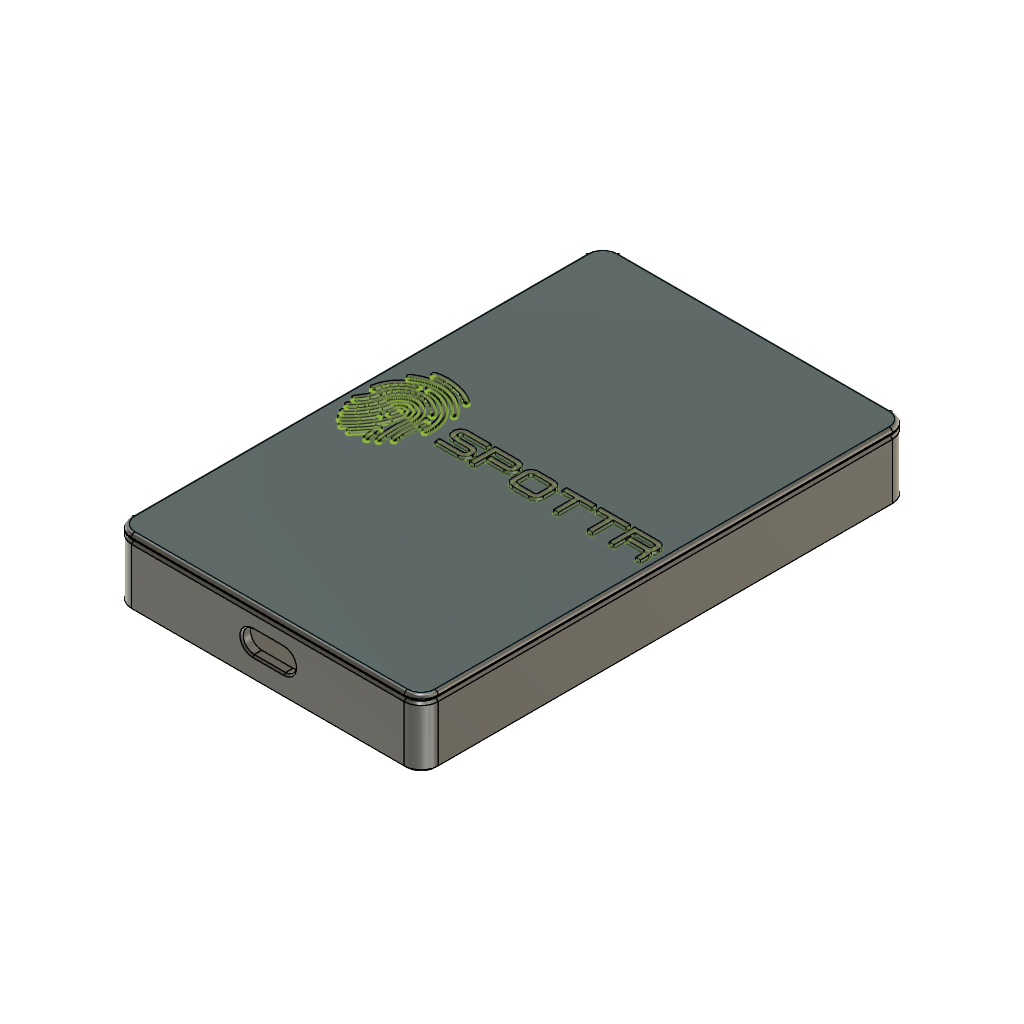
Spottr (Autodesk Fusion 360 archive; units mm, degrees)
design "CASE_BODY"
Autodesk Fusion 360 part; units mm, degrees
note: some values were not read from the file. Set by a fixed rule: which sketch regions a step uses.
(part 1 of 5)
sketch "CARD_SKETCH" plane through (0, 0, 0) normal (0, 0, 1) x (1, 0, 0)
  line L0 (0, 0) -> (54, 0)
  line L1 (54, 0) -> (54, 86)
  line L2 (54, 86) -> (0, 86)
  line L3 (0, 86) -> (0, 0)
  dimension "d3" = 54
  dimension "d4" = 86
  constraint horizontal L0
  constraint vertical L1
  constraint horizontal L2
  constraint vertical L3
  constraint coincident L0.start L3.end
  measures "d3" distance of L0.start L0.end
  measures "d4" distance of L0.start L2.end
extrude "Extrude1" add sketch "CARD_SKETCH" along normal blind 11.9 contours L0 L1 L2 L3 picked at (18, 28.666667) makes body 1
fillet "Fillet1" radius 3 4 edges at (54, 0, 5.95) (0, 0, 5.95) (54, 86, 5.95) (0, 86, 5.95) on bodies 1
ref_plane "WorkPlane1" through (27, 43, 10.7) normal (0, 0, -1) x (-1, 0, 0)
split "Split1" by plane through (27, 43, 10.7) normal (0, 0, -1) bodies 1 makes body 2 at (18, 56.333333, 0)
sketch "CARD_HOLLOW_SKETCH" plane through (0, 0, 10.7) normal (0, 0, 1) x (-1, 0, 0)
  arc A0 (0, -3) -> (-3, 0) centre (-3, -3) ccw
  line L0 (-3, 0) -> (-51, 0)
  arc A1 (-51, 0) -> (-54, -3) centre (-51, -3) ccw
  line L1 (-54, -3) -> (-54, -83)
  arc A2 (-54, -83) -> (-51, -86) centre (-51, -83) ccw
  line L2 (-51, -86) -> (-3, -86)
  arc A3 (-3, -86) -> (0, -83) centre (-3, -83) ccw
  line L3 (0, -83) -> (0, -3)
  line L4 (-54, -83) -> (-54, -3)
  arc A4 (-54, -83) -> (-51, -86) centre (-51, -83) ccw
  line L5 (-3, -86) -> (-51, -86)
  arc A5 (-3, -86) -> (0, -83) centre (-3, -83) ccw
  line L6 (0, -3) -> (0, -83)
  arc A6 (-51, 0) -> (-54, -3) centre (-51, -3) ccw
  line L7 (-51, 0) -> (-3, 0)
  arc A7 (0, -3) -> (-3, 0) centre (-3, -3) ccw
  line L8 (-51, -84.4) -> (-3, -84.4)
  arc A8 (-3, -84.4) -> (-1.6, -83) centre (-3, -83) ccw
  line L9 (-1.6, -83) -> (-1.6, -3)
  arc A9 (-1.6, -3) -> (-3, -1.6) centre (-3, -3) ccw
  line L10 (-3, -1.6) -> (-51, -1.6)
  arc A10 (-51, -1.6) -> (-52.4, -3) centre (-51, -3) ccw
  line L11 (-52.4, -3) -> (-52.4, -83)
  arc A11 (-52.4, -83) -> (-51, -84.4) centre (-51, -83) ccw
extrude "Extrude2" cut sketch "CARD_HOLLOW_SKETCH" against normal blind 9.5 contours L8 A8 L9 A9 L10 A10 L11 A11 picked at (-35.466667, -29.666667) bodies 2
sketch "LID_PLUG_SKETCH" plane through (0, 0, 10.7) normal (0, 0, -1) x (1, 0, 0)
  arc A0 (3, 0) -> (0, -3) centre (3, -3) ccw
  line L0 (0, -3) -> (0, -83)
  arc A1 (0, -83) -> (3, -86) centre (3, -83) ccw
  line L1 (3, -86) -> (51, -86)
  arc A2 (51, -86) -> (54, -83) centre (51, -83) ccw
  line L2 (54, -83) -> (54, -3)
  arc A3 (54, -3) -> (51, 0) centre (51, -3) ccw
  line L3 (51, 0) -> (3, 0)
  line L4 (3, -84.2) -> (51, -84.2)
  arc A4 (51, -84.2) -> (52.2, -83) centre (51, -83) ccw
  line L5 (52.2, -83) -> (52.2, -3)
  arc A5 (52.2, -3) -> (51, -1.8) centre (51, -3) ccw
  line L6 (51, -1.8) -> (3, -1.8)
  arc A6 (3, -1.8) -> (1.8, -3) centre (3, -3) ccw
  line L7 (1.8, -3) -> (1.8, -83)
  arc A7 (1.8, -83) -> (3, -84.2) centre (3, -83) ccw
  line L8 (51.4, -83) -> (51.4, -3)
  arc A8 (51.4, -3) -> (51, -2.6) centre (51, -3) ccw
  line L9 (51, -2.6) -> (3, -2.6)
  arc A9 (3, -2.6) -> (2.6, -3) centre (3, -3) ccw
  line L10 (2.6, -3) -> (2.6, -83)
  arc A10 (2.6, -83) -> (3, -83.4) centre (3, -83) ccw
  line L11 (3, -83.4) -> (51, -83.4)
  arc A11 (51, -83.4) -> (51.4, -83) centre (51, -83) ccw
extrude "Extrude3" add sketch "LID_PLUG_SKETCH" along normal blind 1 contours L4 A4 L5 A5 L6 A6 L7 A7 picked at (51.933333, -56.333333) bodies 1
ref_plane "WorkPlane3" through (27, 43, 5.35) normal (0, 1, 0) x (-1, 0, 0)
chamfer "Chamfer1" distance 0.5 angle 45 1 faces at (18, 56.333333, 0) tangent chain off on bodies 2
chamfer "Chamfer3" distance 0.4 angle 45 8 edges at (0, 43, 10.7) (0.87868, 85.12132, 10.7) (27, 86, 10.7) (53.12132, 85.12132, 10.7) (54, 43, 10.7) (53.12132, 0.87868, 10.7) (27, 0, 10.7) (0.87868, 0.87868, 10.7) tangent chain off on bodies 2
fillet "Fillet2" radius 0.6 1 faces at (18, 56.333333, 11.9) on bodies 1
chamfer "Chamfer4" distance 0.4 angle 45 8 edges at (0, 43, 10.7) (0.87868, 85.12132, 10.7) (27, 86, 10.7) (53.12132, 85.12132, 10.7) (54, 43, 10.7) (53.12132, 0.87868, 10.7) (27, 0, 10.7) (0.87868, 0.87868, 10.7) tangent chain off on bodies 1
sketch "LID_LOGO_SPOTTR_SKETCH" plane through (0, 0, 11.9) normal (0, 0, 1) x (-1, 0, 0)
  arc A0 (-3, -85.4) -> (-0.6, -83) centre (-3, -83) ccw
  line L0 (-0.6, -83) -> (-0.6, -3)
  arc A1 (-0.6, -3) -> (-3, -0.6) centre (-3, -3) ccw
  line L1 (-3, -0.6) -> (-51, -0.6)
  arc A2 (-51, -0.6) -> (-53.4, -3) centre (-51, -3) ccw
  line L2 (-53.4, -3) -> (-53.4, -83)
  arc A3 (-53.4, -83) -> (-51, -85.4) centre (-51, -83) ccw
  line L3 (-51, -85.4) -> (-3, -85.4)
  spline S0 degree 3 poles (-5.943652, -50.073493) (-6.506523, -50.208843) (-7.077484, -50.282586) (-7.656535, -50.294098) knots 0 0 0 0 1 1 1 1
  spline S1 degree 3 poles (-7.656535, -50.294098) (-8.235274, -50.305922) (-8.808724, -50.255515) (-9.376574, -50.142879) knots 0 0 0 0 1 1 1 1
  spline S2 degree 3 poles (-9.376574, -50.142879) (-9.948468, -50.05109) (-10.504182, -49.89956) (-11.043407, -49.688288) knots 0 0 0 0 1 1 1 1
  spline S3 degree 3 poles (-11.043407, -49.688288) (-11.58294, -49.476706) (-12.093539, -49.210362) (-12.575511, -48.888943) knots 0 0 0 0 1 1 1 1
  spline S4 degree 3 poles (-12.575511, -48.888943) (-12.594491, -48.875253) (-12.614716, -48.86374) (-12.635874, -48.854095) knots 0 0 0 0 1 1 1 1
  spline S5 degree 3 poles (-12.635874, -48.854095) (-12.657343, -48.844138) (-12.679435, -48.83667) (-12.702149, -48.831381) knots 0 0 0 0 1 1 1 1
  spline S6 degree 3 poles (-12.702149, -48.831381) (-12.724863, -48.826091) (-12.748199, -48.823291) (-12.771536, -48.822668) knots 0 0 0 0 1 1 1 1
  spline S7 degree 3 poles (-12.771536, -48.822668) (-12.794872, -48.821737) (-12.818208, -48.823599) (-12.841233, -48.827647) knots 0 0 0 0 1 1 1 1
  spline S8 degree 3 poles (-12.841233, -48.827647) (-12.864258, -48.831383) (-12.886661, -48.837604) (-12.908753, -48.846316) knots 0 0 0 0 1 1 1 1
  spline S9 degree 3 poles (-12.908753, -48.846316) (-12.930533, -48.854717) (-12.951069, -48.865296) (-12.970983, -48.877742) knots 0 0 0 0 1 1 1 1
  spline S10 degree 3 poles (-12.970983, -48.877742) (-12.990585, -48.890499) (-13.008943, -48.905123) (-13.025745, -48.921303) knots 0 0 0 0 1 1 1 1
  spline S11 degree 3 poles (-13.025745, -48.921303) (-13.042547, -48.937483) (-13.057794, -48.955218) (-13.070862, -48.974821) knots 0 0 0 0 1 1 1 1
  spline S12 degree 3 poles (-13.070862, -48.974821) (-13.084242, -48.994112) (-13.095443, -49.014337) (-13.104778, -49.035806) knots 0 0 0 0 1 1 1 1
  spline S13 degree 3 poles (-13.104778, -49.035806) (-13.114112, -49.057587) (-13.120957, -49.079679) (-13.125625, -49.102704) knots 0 0 0 0 1 1 1 1
  spline S14 degree 3 poles (-13.125625, -49.102704) (-13.130603, -49.125729) (-13.133089, -49.148754) (-13.133089, -49.172401) knots 0 0 0 0 1 1 1 1
  spline S15 degree 3 poles (-13.133089, -49.172401) (-13.133407, -49.195738) (-13.131224, -49.219074) (-13.126557, -49.242099) knots 0 0 0 0 1 1 1 1
  spline S16 degree 3 poles (-13.126557, -49.242099) (-13.1222, -49.265124) (-13.115355, -49.287216) (-13.106643, -49.308996) knots 0 0 0 0 1 1 1 1
  spline S17 degree 3 poles (-13.106643, -49.308996) (-13.09762, -49.330777) (-13.086418, -49.351313) (-13.073661, -49.370604) knots 0 0 0 0 1 1 1 1
  spline S18 degree 3 poles (-13.073661, -49.370604) (-13.060593, -49.390207) (-13.045658, -49.408253) (-13.028856, -49.424744) knots 0 0 0 0 1 1 1 1
  spline S19 degree 3 poles (-13.028856, -49.424744) (-13.012365, -49.441235) (-12.994318, -49.455859) (-12.974716, -49.468616) knots 0 0 0 0 1 1 1 1
  spline S20 degree 3 poles (-12.974716, -49.468616) (-12.451361, -49.81866) (-11.896891, -50.108964) (-11.310995, -50.339526) knots 0 0 0 0 1 1 1 1
  spline S21 degree 3 poles (-11.310995, -50.339526) (-10.725099, -50.570088) (-10.121779, -50.73562) (-9.500411, -50.836122) knots 0 0 0 0 1 1 1 1
  spline S22 degree 3 poles (-9.500411, -50.836122) (-8.882467, -50.957471) (-8.258611, -51.011611) (-7.629154, -50.997609) knots 0 0 0 0 1 1 1 1
  spline S23 degree 3 poles (-7.629154, -50.997609) (-6.999386, -50.983918) (-6.378641, -50.902708) (-5.766608, -50.754289) knots 0 0 0 0 1 1 1 1
  spline S24 degree 3 poles (-5.766608, -50.754289) (-5.743583, -50.749) (-5.721492, -50.741532) (-5.700022, -50.731887) knots 0 0 0 0 1 1 1 1
  spline S25 degree 3 poles (-5.700022, -50.731887) (-5.678864, -50.722241) (-5.658639, -50.710417) (-5.639348, -50.696415) knots 0 0 0 0 1 1 1 1
  spline S26 degree 3 poles (-5.639348, -50.696415) (-5.620368, -50.682725) (-5.602944, -50.667167) (-5.587075, -50.650054) knots 0 0 0 0 1 1 1 1
  spline S27 degree 3 poles (-5.587075, -50.650054) (-5.570894, -50.63263) (-5.556893, -50.613961) (-5.544758, -50.593736) knots 0 0 0 0 1 1 1 1
  spline S28 degree 3 poles (-5.544758, -50.593736) (-5.532623, -50.573511) (-5.522666, -50.552353) (-5.514577, -50.530261) knots 0 0 0 0 1 1 1 1
  spline S29 degree 3 poles (-5.514577, -50.530261) (-5.506487, -50.508169) (-5.500887, -50.485456) (-5.497464, -50.462119) knots 0 0 0 0 1 1 1 1
  spline S30 degree 3 poles (-5.497464, -50.462119) (-5.494038, -50.438783) (-5.493106, -50.415447) (-5.494349, -50.39211) knots 0 0 0 0 1 1 1 1
  spline S31 degree 3 poles (-5.494349, -50.39211) (-5.495592, -50.368463) (-5.499327, -50.345438) (-5.505239, -50.322724) knots 0 0 0 0 1 1 1 1
  spline S32 degree 3 poles (-5.505239, -50.322724) (-5.51115, -50.299699) (-5.519241, -50.277918) (-5.529509, -50.25676) knots 0 0 0 0 1 1 1 1
  spline S33 degree 3 poles (-5.529509, -50.25676) (-5.539777, -50.235602) (-5.552223, -50.215688) (-5.566536, -50.197019) knots 0 0 0 0 1 1 1 1
  spline S34 degree 3 poles (-5.566536, -50.197019) (-5.580849, -50.17835) (-5.596717, -50.161237) (-5.614454, -50.145991) knots 0 0 0 0 1 1 1 1
  spline S35 degree 3 poles (-5.614454, -50.145991) (-5.632189, -50.130433) (-5.651169, -50.116742) (-5.671705, -50.10523) knots 0 0 0 0 1 1 1 1
  spline S36 degree 3 poles (-5.671705, -50.10523) (-5.692241, -50.093717) (-5.713711, -50.084072) (-5.735802, -50.076915) knots 0 0 0 0 1 1 1 1
  spline S37 degree 3 poles (-5.735802, -50.076915) (-5.758204, -50.069452) (-5.78123, -50.064469) (-5.804566, -50.061669) knots 0 0 0 0 1 1 1 1
  spline S38 degree 3 poles (-5.804566, -50.061669) (-5.827902, -50.059184) (-5.851238, -50.058555) (-5.874575, -50.060738) knots 0 0 0 0 1 1 1 1
  spline S39 degree 3 poles (-5.874575, -50.060738) (-5.897911, -50.062602) (-5.920936, -50.066958) (-5.943652, -50.073493) knots 0 0 0 0 1 1 1 1
  spline S40 degree 3 poles (-4.178186, -47.601092) (-4.26593, -47.6655) (-4.35523, -47.728042) (-4.446086, -47.788094) knots 0 0 0 0 1 1 1 1
  spline S41 degree 3 poles (-4.446086, -47.788094) (-4.536942, -47.848146) (-4.629354, -47.905708) (-4.723321, -47.961093) knots 0 0 0 0 1 1 1 1
  spline S42 degree 3 poles (-4.723321, -47.961093) (-4.816977, -48.016478) (-4.912189, -48.069685) (-5.008646, -48.120091) knots 0 0 0 0 1 1 1 1
  spline S43 degree 3 poles (-5.008646, -48.120091) (-5.105102, -48.170809) (-5.202804, -48.218726) (-5.30175, -48.264465) knots 0 0 0 0 1 1 1 1
  spline S44 degree 3 poles (-5.30175, -48.264465) (-5.400695, -48.309893) (-5.500574, -48.353143) (-5.601698, -48.393592) knots 0 0 0 0 1 1 1 1
  spline S45 degree 3 poles (-5.601698, -48.393592) (-5.702822, -48.434042) (-5.804879, -48.472002) (-5.90787, -48.507473) knots 0 0 0 0 1 1 1 1
  spline S46 degree 3 poles (-5.90787, -48.507473) (-6.010861, -48.542944) (-6.114785, -48.575615) (-6.219332, -48.605797) knots 0 0 0 0 1 1 1 1
  spline S47 degree 3 poles (-6.219332, -48.605797) (-6.323878, -48.635667) (-6.429358, -48.663048) (-6.53546, -48.68794) knots 0 0 0 0 1 1 1 1
  spline S48 degree 3 poles (-6.53546, -48.68794) (-6.641563, -48.712521) (-6.747976, -48.734613) (-6.855322, -48.753904) knots 0 0 0 0 1 1 1 1
  spline S49 degree 3 poles (-6.855322, -48.753904) (-6.962358, -48.773507) (-7.070016, -48.789998) (-7.177985, -48.803688) knots 0 0 0 0 1 1 1 1
  spline S50 degree 3 poles (-7.177985, -48.803688) (-7.285954, -48.81769) (-7.394235, -48.828891) (-7.502827, -48.837292) knots 0 0 0 0 1 1 1 1
  spline S51 degree 3 poles (-7.502827, -48.837292) (-7.611418, -48.845694) (-7.720009, -48.851294) (-7.828912, -48.854095) knots 0 0 0 0 1 1 1 1
  spline S52 degree 3 poles (-7.828912, -48.854095) (-7.937815, -48.856897) (-8.046406, -48.857209) (-8.155309, -48.854413) knots 0 0 0 0 1 1 1 1
  spline S53 degree 3 poles (-8.155309, -48.854413) (-8.264211, -48.851929) (-8.372803, -48.846323) (-8.481394, -48.838233) knots 0 0 0 0 1 1 1 1
  spline S54 degree 3 poles (-8.481394, -48.838233) (-8.589986, -48.830143) (-8.698266, -48.818942) (-8.806235, -48.805562) knots 0 0 0 0 1 1 1 1
  spline S55 degree 3 poles (-8.806235, -48.805562) (-8.914204, -48.791872) (-9.021862, -48.775381) (-9.129209, -48.75609) knots 0 0 0 0 1 1 1 1
  spline S56 degree 3 poles (-9.129209, -48.75609) (-9.236245, -48.737109) (-9.342969, -48.715329) (-9.449072, -48.690748) knots 0 0 0 0 1 1 1 1
  spline S57 degree 3 poles (-9.449072, -48.690748) (-9.555174, -48.666167) (-9.660343, -48.639097) (-9.7652, -48.609227) knots 0 0 0 0 1 1 1 1
  spline S58 degree 3 poles (-9.7652, -48.609227) (-9.869747, -48.579356) (-9.973671, -48.546685) (-10.076662, -48.511525) knots 0 0 0 0 1 1 1 1
  spline S59 degree 3 poles (-10.076662, -48.511525) (-10.179652, -48.476365) (-10.28171, -48.438716) (-10.382834, -48.398267) knots 0 0 0 0 1 1 1 1
  spline S60 degree 3 poles (-10.382834, -48.398267) (-10.483957, -48.357817) (-10.584148, -48.31519) (-10.683094, -48.269762) knots 0 0 0 0 1 1 1 1
  spline S61 degree 3 poles (-10.683094, -48.269762) (-10.782039, -48.224334) (-10.879741, -48.176417) (-10.976197, -48.12601) knots 0 0 0 0 1 1 1 1
  spline S62 degree 3 poles (-10.976197, -48.12601) (-11.072965, -48.075604) (-11.167866, -48.022708) (-11.261833, -47.967635) knots 0 0 0 0 1 1 1 1
  spline S63 degree 3 poles (-11.261833, -47.967635) (-11.355801, -47.91225) (-11.448212, -47.854687) (-11.539068, -47.794946) knots 0 0 0 0 1 1 1 1
  spline S64 degree 3 poles (-11.539068, -47.794946) (-11.629924, -47.734894) (-11.719224, -47.672664) (-11.80728, -47.608256) knots 0 0 0 0 1 1 1 1
  spline S65 degree 3 poles (-11.80728, -47.608256) (-11.895024, -47.543848) (-11.980901, -47.477262) (-12.065534, -47.408498) knots 0 0 0 0 1 1 1 1
  spline S66 degree 3 poles (-12.065534, -47.408498) (-12.149856, -47.339733) (-12.232311, -47.268791) (-12.31321, -47.195671) knots 0 0 0 0 1 1 1 1
  spline S67 degree 3 poles (-12.31321, -47.195671) (-12.394109, -47.122862) (-12.473141, -47.047874) (-12.549995, -46.970709) knots 0 0 0 0 1 1 1 1
  spline S68 degree 3 poles (-12.549995, -46.970709) (-12.627161, -46.893855) (-12.702148, -46.814823) (-12.775268, -46.733924) knots 0 0 0 0 1 1 1 1
  spline S69 degree 3 poles (-12.775268, -46.733924) (-12.848077, -46.653336) (-12.91902, -46.57057) (-12.988095, -46.486248) knots 0 0 0 0 1 1 1 1
  spline S70 degree 3 poles (-12.988095, -46.486248) (-13.056859, -46.401615) (-13.123445, -46.315738) (-13.187853, -46.227682) knots 0 0 0 0 1 1 1 1
  spline S71 degree 3 poles (-13.187853, -46.227682) (-13.252573, -46.139938) (-13.314803, -46.050638) (-13.374544, -45.959782) knots 0 0 0 0 1 1 1 1
  spline S72 degree 3 poles (-13.374544, -45.959782) (-13.401614, -45.923066) (-13.434596, -45.893196) (-13.473489, -45.869548) knots 0 0 0 0 1 1 1 1
  spline S73 degree 3 poles (-13.473489, -45.869548) (-13.512072, -45.845901) (-13.553766, -45.830343) (-13.598572, -45.822876) knots 0 0 0 0 1 1 1 1
  spline S74 degree 3 poles (-13.598572, -45.822876) (-13.643377, -45.815413) (-13.687872, -45.816344) (-13.732366, -45.826301) knots 0 0 0 0 1 1 1 1
  spline S75 degree 3 poles (-13.732366, -45.826301) (-13.77655, -45.835946) (-13.81731, -45.853682) (-13.85496, -45.879508) knots 0 0 0 0 1 1 1 1
  spline S76 degree 3 poles (-13.85496, -45.879508) (-13.892298, -45.905022) (-13.923724, -45.936759) (-13.948927, -45.97472) knots 0 0 0 0 1 1 1 1
  spline S77 degree 3 poles (-13.948927, -45.97472) (-13.97413, -46.012369) (-13.991244, -46.053441) (-14.000578, -46.097935) knots 0 0 0 0 1 1 1 1
  spline S78 degree 3 poles (-14.000578, -46.097935) (-14.009913, -46.14243) (-14.010535, -46.187235) (-14.002752, -46.23173) knots 0 0 0 0 1 1 1 1
  spline S79 degree 3 poles (-14.002752, -46.23173) (-13.994663, -46.276535) (-13.978794, -46.318229) (-13.954524, -46.356812) knots 0 0 0 0 1 1 1 1
  spline S80 degree 3 poles (-13.954524, -46.356812) (-13.888249, -46.457314) (-13.819174, -46.555948) (-13.747609, -46.653027) knots 0 0 0 0 1 1 1 1
  spline S81 degree 3 poles (-13.747609, -46.653027) (-13.676045, -46.750106) (-13.601991, -46.845318) (-13.525759, -46.938663) knots 0 0 0 0 1 1 1 1
  spline S82 degree 3 poles (-13.525759, -46.938663) (-13.449527, -47.032008) (-13.370806, -47.123175) (-13.289907, -47.212475) knots 0 0 0 0 1 1 1 1
  spline S83 degree 3 poles (-13.289907, -47.212475) (-13.209008, -47.302087) (-13.125931, -47.389209) (-13.040365, -47.474153) knots 0 0 0 0 1 1 1 1
  spline S84 degree 3 poles (-13.040365, -47.474153) (-12.955109, -47.559408) (-12.867676, -47.642174) (-12.778065, -47.723073) knots 0 0 0 0 1 1 1 1
  spline S85 degree 3 poles (-12.778065, -47.723073) (-12.688765, -47.803661) (-12.596975, -47.882071) (-12.50363, -47.957991) knots 0 0 0 0 1 1 1 1
  spline S86 degree 3 poles (-12.50363, -47.957991) (-12.409974, -48.034223) (-12.314762, -48.107655) (-12.217683, -48.178908) knots 0 0 0 0 1 1 1 1
  spline S87 degree 3 poles (-12.217683, -48.178908) (-12.120293, -48.250162) (-12.021347, -48.318926) (-11.920535, -48.385201) knots 0 0 0 0 1 1 1 1
  spline S88 degree 3 poles (-11.920535, -48.385201) (-11.820034, -48.451165) (-11.717665, -48.51495) (-11.613741, -48.575936) knots 0 0 0 0 1 1 1 1
  spline S89 degree 3 poles (-11.613741, -48.575936) (-11.509816, -48.636921) (-11.404648, -48.695418) (-11.297612, -48.750802) knots 0 0 0 0 1 1 1 1
  spline S90 degree 3 poles (-11.297612, -48.750802) (-11.190887, -48.806498) (-11.082607, -48.859705) (-10.973082, -48.9098) knots 0 0 0 0 1 1 1 1
  spline S91 degree 3 poles (-10.973082, -48.9098) (-10.863557, -48.959895) (-10.752788, -49.007501) (-10.640774, -49.051996) knots 0 0 0 0 1 1 1 1
  spline S92 degree 3 poles (-10.640774, -49.051996) (-10.529071, -49.09649) (-10.415812, -49.138185) (-10.301931, -49.177078) knots 0 0 0 0 1 1 1 1
  spline S93 degree 3 poles (-10.301931, -49.177078) (-10.187739, -49.215972) (-10.072924, -49.252066) (-9.957176, -49.285047) knots 0 0 0 0 1 1 1 1
  spline S94 degree 3 poles (-9.957176, -49.285047) (-9.841117, -49.318029) (-9.724747, -49.348211) (-9.607132, -49.375281) knots 0 0 0 0 1 1 1 1
  spline S95 degree 3 poles (-9.607132, -49.375281) (-9.489829, -49.402351) (-9.371903, -49.426621) (-9.253354, -49.447779) knots 0 0 0 0 1 1 1 1
  spline S96 degree 3 poles (-9.253354, -49.447779) (-9.134495, -49.468937) (-9.015636, -49.486984) (-8.896154, -49.50223) knots 0 0 0 0 1 1 1 1
  spline S97 degree 3 poles (-8.896154, -49.50223) (-8.776672, -49.517477) (-8.656568, -49.529612) (-8.536464, -49.538635) knots 0 0 0 0 1 1 1 1
  spline S98 degree 3 poles (-8.536464, -49.538635) (-8.41636, -49.547658) (-8.296256, -49.55357) (-8.17553, -49.556682) knots 0 0 0 0 1 1 1 1
  spline S99 degree 3 poles (-8.17553, -49.556682) (-8.055115, -49.559484) (-7.9347, -49.559484) (-7.814284, -49.556363) knots 0 0 0 0 1 1 1 1
  spline S100 degree 3 poles (-7.814284, -49.556363) (-7.693869, -49.553249) (-7.573765, -49.547029) (-7.45335, -49.538005) knots 0 0 0 0 1 1 1 1
  spline S101 degree 3 poles (-7.45335, -49.538005) (-7.333246, -49.528671) (-7.213454, -49.516536) (-7.093972, -49.50129) knots 0 0 0 0 1 1 1 1
  spline S102 degree 3 poles (-7.093972, -49.50129) (-6.97449, -49.486043) (-6.855319, -49.467685) (-6.736771, -49.446216) knots 0 0 0 0 1 1 1 1
  spline S103 degree 3 poles (-6.736771, -49.446216) (-6.618223, -49.425058) (-6.500297, -49.400788) (-6.382993, -49.373407) knots 0 0 0 0 1 1 1 1
  spline S104 degree 3 poles (-6.382993, -49.373407) (-6.265378, -49.346026) (-6.149008, -49.315844) (-6.032949, -49.282862) knots 0 0 0 0 1 1 1 1
  spline S105 degree 3 poles (-6.032949, -49.282862) (-5.917202, -49.249569) (-5.802387, -49.213476) (-5.688195, -49.174271) knots 0 0 0 0 1 1 1 1
  spline S106 degree 3 poles (-5.688195, -49.174271) (-5.574314, -49.135377) (-5.461055, -49.093683) (-5.349352, -49.048877) knots 0 0 0 0 1 1 1 1
  spline S107 degree 3 poles (-5.349352, -49.048877) (-5.237338, -49.004071) (-5.126568, -48.956465) (-5.017043, -48.90637) knots 0 0 0 0 1 1 1 1
  spline S108 degree 3 poles (-5.017043, -48.90637) (-4.907518, -48.855964) (-4.799549, -48.802757) (-4.692514, -48.747061) knots 0 0 0 0 1 1 1 1
  spline S109 degree 3 poles (-4.692514, -48.747061) (-4.585789, -48.691365) (-4.480309, -48.632869) (-4.376385, -48.571573) knots 0 0 0 0 1 1 1 1
  spline S110 degree 3 poles (-4.376385, -48.571573) (-4.272461, -48.510587) (-4.170403, -48.446801) (-4.069591, -48.380526) knots 0 0 0 0 1 1 1 1
  spline S111 degree 3 poles (-4.069591, -48.380526) (-3.969089, -48.31394) (-3.870143, -48.245176) (-3.772753, -48.173922) knots 0 0 0 0 1 1 1 1
  spline S112 degree 3 poles (-3.772753, -48.173922) (-3.738216, -48.145608) (-3.709901, -48.112004) (-3.68812, -48.07311) knots 0 0 0 0 1 1 1 1
  spline S113 degree 3 poles (-3.68812, -48.07311) (-3.66634, -48.034216) (-3.652338, -47.992833) (-3.646426, -47.948339) knots 0 0 0 0 1 1 1 1
  spline S114 degree 3 poles (-3.646426, -47.948339) (-3.640514, -47.904155) (-3.642693, -47.860594) (-3.653272, -47.817033) knots 0 0 0 0 1 1 1 1
  spline S115 degree 3 poles (-3.653272, -47.817033) (-3.663851, -47.773783) (-3.682209, -47.733956) (-3.708034, -47.697551) knots 0 0 0 0 1 1 1 1
  spline S116 degree 3 poles (-3.708034, -47.697551) (-3.733548, -47.661147) (-3.765286, -47.630654) (-3.802624, -47.606384) knots 0 0 0 0 1 1 1 1
  spline S117 degree 3 poles (-3.802624, -47.606384) (-3.839962, -47.581803) (-3.880411, -47.565313) (-3.923972, -47.556289) knots 0 0 0 0 1 1 1 1
  spline S118 degree 3 poles (-3.923972, -47.556289) (-3.967844, -47.547266) (-4.011406, -47.546643) (-4.055278, -47.554425) knots 0 0 0 0 1 1 1 1
  spline S119 degree 3 poles (-4.055278, -47.554425) (-4.09915, -47.562206) (-4.140222, -47.577761) (-4.178186, -47.601092) knots 0 0 0 0 1 1 1 1
  spline S120 degree 3 poles (-9.005682, -48.063773) (-8.513443, -48.151828) (-8.018091, -48.177654) (-7.519629, -48.140938) knots 0 0 0 0 1 1 1 1
  spline S121 degree 3 poles (-7.519629, -48.140938) (-7.496294, -48.139696) (-7.473267, -48.136271) (-7.450553, -48.13067) knots 0 0 0 0 1 1 1 1
  spline S122 degree 3 poles (-7.450553, -48.13067) (-7.427839, -48.124761) (-7.405748, -48.11698) (-7.384901, -48.106712) knots 0 0 0 0 1 1 1 1
  spline S123 degree 3 poles (-7.384901, -48.106712) (-7.363742, -48.096444) (-7.343828, -48.084309) (-7.32516, -48.070307) knots 0 0 0 0 1 1 1 1
  spline S124 degree 3 poles (-7.32516, -48.070307) (-7.30649, -48.055994) (-7.289377, -48.040125) (-7.27382, -48.022701) knots 0 0 0 0 1 1 1 1
  spline S125 degree 3 poles (-7.27382, -48.022701) (-7.258262, -48.005277) (-7.244572, -47.986296) (-7.232747, -47.966072) knots 0 0 0 0 1 1 1 1
  spline S126 degree 3 poles (-7.232747, -47.966072) (-7.220924, -47.945536) (-7.211278, -47.924378) (-7.203811, -47.902286) knots 0 0 0 0 1 1 1 1
  spline S127 degree 3 poles (-7.203811, -47.902286) (-7.196347, -47.879883) (-7.191054, -47.857169) (-7.188253, -47.833833) knots 0 0 0 0 1 1 1 1
  spline S128 degree 3 poles (-7.188253, -47.833833) (-7.185138, -47.810808) (-7.184517, -47.787471) (-7.186079, -47.764135) knots 0 0 0 0 1 1 1 1
  spline S129 degree 3 poles (-7.186079, -47.764135) (-7.187942, -47.740488) (-7.191989, -47.717463) (-7.198213, -47.69506) knots 0 0 0 0 1 1 1 1
  spline S130 degree 3 poles (-7.198213, -47.69506) (-7.204435, -47.672346) (-7.212838, -47.650565) (-7.223417, -47.629718) knots 0 0 0 0 1 1 1 1
  spline S131 degree 3 poles (-7.223417, -47.629718) (-7.233996, -47.608871) (-7.246752, -47.589269) (-7.261065, -47.570911) knots 0 0 0 0 1 1 1 1
  spline S132 degree 3 poles (-7.261065, -47.570911) (-7.27569, -47.552553) (-7.291869, -47.535751) (-7.309916, -47.520504) knots 0 0 0 0 1 1 1 1
  spline S133 degree 3 poles (-7.309916, -47.520504) (-7.327651, -47.505569) (-7.346943, -47.49219) (-7.367479, -47.480988) knots 0 0 0 0 1 1 1 1
  spline S134 degree 3 poles (-7.367479, -47.480988) (-7.388015, -47.469476) (-7.409173, -47.460452) (-7.431576, -47.453607) knots 0 0 0 0 1 1 1 1
  spline S135 degree 3 poles (-7.431576, -47.453607) (-7.453978, -47.446453) (-7.476692, -47.441783) (-7.500029, -47.439294) knots 0 0 0 0 1 1 1 1
  spline S136 degree 3 poles (-7.500029, -47.439294) (-7.523365, -47.43681) (-7.546701, -47.43681) (-7.570037, -47.438976) knots 0 0 0 0 1 1 1 1
  spline S137 degree 3 poles (-7.570037, -47.438976) (-7.669606, -47.44613) (-7.769485, -47.450488) (-7.869675, -47.452044) knots 0 0 0 0 1 1 1 1
  spline S138 degree 3 poles (-7.869675, -47.452044) (-7.969554, -47.453597) (-8.069434, -47.452363) (-8.169312, -47.447997) knots 0 0 0 0 1 1 1 1
  spline S139 degree 3 poles (-8.169312, -47.447997) (-8.269191, -47.443949) (-8.36907, -47.436795) (-8.468327, -47.42715) knots 0 0 0 0 1 1 1 1
  spline S140 degree 3 poles (-8.468327, -47.42715) (-8.567895, -47.417193) (-8.667152, -47.404436) (-8.765787, -47.388878) knots 0 0 0 0 1 1 1 1
  spline S141 degree 3 poles (-8.765787, -47.388878) (-8.864733, -47.373632) (-8.962745, -47.355274) (-9.060445, -47.334116) knots 0 0 0 0 1 1 1 1
  spline S142 degree 3 poles (-9.060445, -47.334116) (-9.158146, -47.312957) (-9.255225, -47.28931) (-9.351682, -47.262551) knots 0 0 0 0 1 1 1 1
  spline S143 degree 3 poles (-9.351682, -47.262551) (-9.448138, -47.236103) (-9.543661, -47.206855) (-9.638251, -47.174807) knots 0 0 0 0 1 1 1 1
  spline S144 degree 3 poles (-9.638251, -47.174807) (-9.733152, -47.142758) (-9.826808, -47.107909) (-9.919531, -47.070571) knots 0 0 0 0 1 1 1 1
  spline S145 degree 3 poles (-9.919531, -47.070571) (-10.012254, -47.033233) (-10.103732, -46.993095) (-10.194277, -46.950779) knots 0 0 0 0 1 1 1 1
  spline S146 degree 3 poles (-10.194277, -46.950779) (-10.284821, -46.908151) (-10.37381, -46.863034) (-10.461866, -46.815428) knots 0 0 0 0 1 1 1 1
  spline S147 degree 3 poles (-10.461866, -46.815428) (-10.54961, -46.767511) (-10.63611, -46.717416) (-10.721365, -46.664831) knots 0 0 0 0 1 1 1 1
  spline S148 degree 3 poles (-10.721365, -46.664831) (-10.806309, -46.612247) (-10.889697, -46.557485) (-10.971841, -46.500233) knots 0 0 0 0 1 1 1 1
  spline S149 degree 3 poles (-10.971841, -46.500233) (-11.053674, -46.44267) (-11.13395, -46.38324) (-11.21236, -46.321322) knots 0 0 0 0 1 1 1 1
  spline S150 degree 3 poles (-11.21236, -46.321322) (-11.291081, -46.259403) (-11.367624, -46.195306) (-11.442611, -46.129031) knots 0 0 0 0 1 1 1 1
  spline S151 degree 3 poles (-11.442611, -46.129031) (-11.517599, -46.062756) (-11.590719, -45.994303) (-11.661661, -45.923983) knots 0 0 0 0 1 1 1 1
  spline S152 degree 3 poles (-11.661661, -45.923983) (-11.732604, -45.853663) (-11.801679, -45.781165) (-11.868576, -45.7068) knots 0 0 0 0 1 1 1 1
  spline S153 degree 3 poles (-11.868576, -45.7068) (-11.935474, -45.632435) (-12.000193, -45.556514) (-12.062734, -45.478415) knots 0 0 0 0 1 1 1 1
  spline S154 degree 3 poles (-12.062734, -45.478415) (-12.125586, -45.400317) (-12.185638, -45.320662) (-12.243823, -45.239141) knots 0 0 0 0 1 1 1 1
  spline S155 degree 3 poles (-12.243823, -45.239141) (-12.302009, -45.157619) (-12.357704, -45.074542) (-12.410911, -44.989909) knots 0 0 0 0 1 1 1 1
  spline S156 degree 3 poles (-12.410911, -44.989909) (-12.464429, -44.905277) (-12.515147, -44.819088) (-12.563686, -44.731655) knots 0 0 0 0 1 1 1 1
  spline S157 degree 3 poles (-12.563686, -44.731655) (-12.612225, -44.644221) (-12.658276, -44.555232) (-12.701526, -44.46531) knots 0 0 0 0 1 1 1 1
  spline S158 degree 3 poles (-12.701526, -44.46531) (-12.745087, -44.375076) (-12.785847, -44.283598) (-12.824119, -44.191187) knots 0 0 0 0 1 1 1 1
  spline S159 degree 3 poles (-12.824119, -44.191187) (-12.86239, -44.098775) (-12.897863, -44.005119) (-12.930843, -43.91084) knots 0 0 0 0 1 1 1 1
  spline S160 degree 3 poles (-12.930843, -43.91084) (-12.963825, -43.816251) (-12.994007, -43.721039) (-13.021699, -43.624582) knots 0 0 0 0 1 1 1 1
  spline S161 degree 3 poles (-13.021699, -43.624582) (-13.04908, -43.528437) (-13.073972, -43.431669) (-13.096064, -43.333968) knots 0 0 0 0 1 1 1 1
  spline S162 degree 3 poles (-13.096064, -43.333968) (-13.118156, -43.236266) (-13.137136, -43.137943) (-13.153627, -43.039308) knots 0 0 0 0 1 1 1 1
  spline S163 degree 3 poles (-13.153627, -43.039308) (-13.170118, -42.940674) (-13.183809, -42.841417) (-13.194699, -42.741849) knots 0 0 0 0 1 1 1 1
  spline S164 degree 3 poles (-13.194699, -42.741849) (-13.205589, -42.64228) (-13.213368, -42.542712) (-13.218657, -42.442833) knots 0 0 0 0 1 1 1 1
  spline S165 degree 3 poles (-13.218657, -42.442833) (-13.223947, -42.342643) (-13.226121, -42.242764) (-13.22581, -42.142573) knots 0 0 0 0 1 1 1 1
  spline S166 degree 3 poles (-13.22581, -42.142573) (-13.225173, -42.042383) (-13.221764, -41.942504) (-13.215542, -41.842624) knots 0 0 0 0 1 1 1 1
  spline S167 degree 3 poles (-13.215542, -41.842624) (-13.209632, -41.742745) (-13.200607, -41.642866) (-13.188783, -41.543609) knots 0 0 0 0 1 1 1 1
  spline S168 degree 3 poles (-13.188783, -41.543609) (-13.17696, -41.444041) (-13.162024, -41.345095) (-13.1446, -41.24646) knots 0 0 0 0 1 1 1 1
  spline S169 degree 3 poles (-13.1446, -41.24646) (-13.140554, -41.223746) (-13.139, -41.200721) (-13.13931, -41.177696) knots 0 0 0 0 1 1 1 1
  spline S170 degree 3 poles (-13.13931, -41.177696) (-13.139629, -41.154671) (-13.142424, -41.131646) (-13.1474, -41.109243) knots 0 0 0 0 1 1 1 1
  spline S171 degree 3 poles (-13.1474, -41.109243) (-13.152379, -41.086529) (-13.159535, -41.064749) (-13.168558, -41.04359) knots 0 0 0 0 1 1 1 1
  spline S172 degree 3 poles (-13.168558, -41.04359) (-13.177893, -41.022432) (-13.189094, -41.002207) (-13.202474, -40.983538) knots 0 0 0 0 1 1 1 1
  spline S173 degree 3 poles (-13.202474, -40.983538) (-13.215542, -40.964558) (-13.230477, -40.946823) (-13.246968, -40.930954) knots 0 0 0 0 1 1 1 1
  spline S174 degree 3 poles (-13.246968, -40.930954) (-13.26377, -40.915085) (-13.281817, -40.900772) (-13.301109, -40.888326) knots 0 0 0 0 1 1 1 1
  spline S175 degree 3 poles (-13.301109, -40.888326) (-13.320711, -40.87588) (-13.341247, -40.865301) (-13.362716, -40.8569) knots 0 0 0 0 1 1 1 1
  spline S176 degree 3 poles (-13.362716, -40.8569) (-13.384186, -40.848499) (-13.406277, -40.842276) (-13.428991, -40.838231) knots 0 0 0 0 1 1 1 1
  spline S177 degree 3 poles (-13.428991, -40.838231) (-13.451705, -40.834184) (-13.474419, -40.832322) (-13.497757, -40.832942) knots 0 0 0 0 1 1 1 1
  spline S178 degree 3 poles (-13.497757, -40.832942) (-13.520782, -40.83326) (-13.543495, -40.836056) (-13.565897, -40.841031) knots 0 0 0 0 1 1 1 1
  spline S179 degree 3 poles (-13.565897, -40.841031) (-13.588611, -40.84601) (-13.610392, -40.853166) (-13.63155, -40.86219) knots 0 0 0 0 1 1 1 1
  spline S180 degree 3 poles (-13.63155, -40.86219) (-13.652708, -40.871524) (-13.672933, -40.882726) (-13.691602, -40.896105) knots 0 0 0 0 1 1 1 1
  spline S181 degree 3 poles (-13.691602, -40.896105) (-13.710582, -40.909173) (-13.728007, -40.924109) (-13.744187, -40.940911) knots 0 0 0 0 1 1 1 1
  spline S182 degree 3 poles (-13.744187, -40.940911) (-13.760054, -40.957713) (-13.774368, -40.97576) (-13.786814, -40.995051) knots 0 0 0 0 1 1 1 1
  spline S183 degree 3 poles (-13.786814, -40.995051) (-13.79926, -41.014653) (-13.809528, -41.035189) (-13.81824, -41.056659) knots 0 0 0 0 1 1 1 1
  spline S184 degree 3 poles (-13.81824, -41.056659) (-13.826641, -41.078128) (-13.832864, -41.10022) (-13.836909, -41.122934) knots 0 0 0 0 1 1 1 1
  spline S185 degree 3 poles (-13.836909, -41.122934) (-13.854023, -41.21939) (-13.868647, -41.316158) (-13.881093, -41.413237) knots 0 0 0 0 1 1 1 1
  spline S186 degree 3 poles (-13.881093, -41.413237) (-13.893228, -41.510316) (-13.903184, -41.607706) (-13.910963, -41.705407) knots 0 0 0 0 1 1 1 1
  spline S187 degree 3 poles (-13.910963, -41.705407) (-13.918427, -41.803108) (-13.92372, -41.900809) (-13.926521, -41.998511) knots 0 0 0 0 1 1 1 1
  spline S188 degree 3 poles (-13.926521, -41.998511) (-13.929325, -42.096523) (-13.929635, -42.194224) (-13.927763, -42.292236) knots 0 0 0 0 1 1 1 1
  spline S189 degree 3 poles (-13.927763, -42.292236) (-13.925588, -42.389938) (-13.921231, -42.48795) (-13.914383, -42.58534) knots 0 0 0 0 1 1 1 1
  spline S190 degree 3 poles (-13.914383, -42.58534) (-13.907852, -42.683041) (-13.898516, -42.780431) (-13.887002, -42.877821) knots 0 0 0 0 1 1 1 1
  spline S191 degree 3 poles (-13.887002, -42.877821) (-13.87549, -42.9749) (-13.861488, -43.071979) (-13.845308, -43.168436) knots 0 0 0 0 1 1 1 1
  spline S192 degree 3 poles (-13.845308, -43.168436) (-13.828817, -43.264892) (-13.810459, -43.361038) (-13.789301, -43.456561) knots 0 0 0 0 1 1 1 1
  spline S193 degree 3 poles (-13.789301, -43.456561) (-13.768454, -43.552084) (-13.745118, -43.647296) (-13.719292, -43.741574) knots 0 0 0 0 1 1 1 1
  spline S194 degree 3 poles (-13.719292, -43.741574) (-13.693778, -43.836164) (-13.665774, -43.92982) (-13.635591, -44.022854) knots 0 0 0 0 1 1 1 1
  spline S195 degree 3 poles (-13.635591, -44.022854) (-13.60541, -44.115888) (-13.572739, -44.2083) (-13.53789, -44.299778) knots 0 0 0 0 1 1 1 1
  spline S196 degree 3 poles (-13.53789, -44.299778) (-13.503353, -44.391256) (-13.466326, -44.481801) (-13.427121, -44.571412) knots 0 0 0 0 1 1 1 1
  spline S197 degree 3 poles (-13.427121, -44.571412) (-13.387916, -44.661024) (-13.346533, -44.749701) (-13.302972, -44.837446) knots 0 0 0 0 1 1 1 1
  spline S198 degree 3 poles (-13.302972, -44.837446) (-13.259411, -44.92519) (-13.213672, -45.01169) (-13.166066, -45.096945) knots 0 0 0 0 1 1 1 1
  spline S199 degree 3 poles (-13.166066, -45.096945) (-13.118149, -45.182511) (-13.068364, -45.266522) (-13.016402, -45.349599) knots 0 0 0 0 1 1 1 1
  spline S200 degree 3 poles (-13.016402, -45.349599) (-12.964751, -45.432365) (-12.910611, -45.514198) (-12.854915, -45.594474) knots 0 0 0 0 1 1 1 1
  spline S201 degree 3 poles (-12.854915, -45.594474) (-12.798908, -45.674751) (-12.741034, -45.753472) (-12.681293, -45.830949) knots 0 0 0 0 1 1 1 1
  spline S202 degree 3 poles (-12.681293, -45.830949) (-12.621553, -45.908425) (-12.559945, -45.984346) (-12.49647, -46.058711) knots 0 0 0 0 1 1 1 1
  spline S203 degree 3 poles (-12.49647, -46.058711) (-12.432996, -46.133387) (-12.367965, -46.206196) (-12.300757, -46.277138) knots 0 0 0 0 1 1 1 1
  spline S204 degree 3 poles (-12.300757, -46.277138) (-12.233859, -46.348392) (-12.165095, -46.418089) (-12.094464, -46.48592) knots 0 0 0 0 1 1 1 1
  spline S205 degree 3 poles (-12.094464, -46.48592) (-12.024144, -46.553751) (-11.951957, -46.619715) (-11.878215, -46.684123) knots 0 0 0 0 1 1 1 1
  spline S206 degree 3 poles (-11.878215, -46.684123) (-11.804783, -46.748531) (-11.729485, -46.810761) (-11.652631, -46.871435) knots 0 0 0 0 1 1 1 1
  spline S207 degree 3 poles (-11.652631, -46.871435) (-11.576088, -46.93211) (-11.497678, -46.990917) (-11.418023, -47.047546) knots 0 0 0 0 1 1 1 1
  spline S208 degree 3 poles (-11.418023, -47.047546) (-11.33868, -47.104487) (-11.25747, -47.159249) (-11.175326, -47.211834) knots 0 0 0 0 1 1 1 1
  spline S209 degree 3 poles (-11.175326, -47.211834) (-11.092871, -47.264729) (-11.009482, -47.315447) (-10.924539, -47.364297) knots 0 0 0 0 1 1 1 1
  spline S210 degree 3 poles (-10.924539, -47.364297) (-10.839906, -47.412837) (-10.754029, -47.459509) (-10.666907, -47.504004) knots 0 0 0 0 1 1 1 1
  spline S211 degree 3 poles (-10.666907, -47.504004) (-10.579784, -47.548498) (-10.491729, -47.590815) (-10.402429, -47.630953) knots 0 0 0 0 1 1 1 1
  spline S212 degree 3 poles (-10.402429, -47.630953) (-10.31344, -47.671091) (-10.223206, -47.709052) (-10.13235, -47.744834) knots 0 0 0 0 1 1 1 1
  spline S213 degree 3 poles (-10.13235, -47.744834) (-10.041182, -47.780616) (-9.949394, -47.813909) (-9.856671, -47.845024) knots 0 0 0 0 1 1 1 1
  spline S214 degree 3 poles (-9.856671, -47.845024) (-9.76426, -47.876451) (-9.670914, -47.905388) (-9.576636, -47.931835) knots 0 0 0 0 1 1 1 1
  spline S215 degree 3 poles (-9.576636, -47.931835) (-9.482669, -47.958594) (-9.388079, -47.982864) (-9.292867, -48.004956) knots 0 0 0 0 1 1 1 1
  spline S216 degree 3 poles (-9.292867, -48.004956) (-9.197344, -48.027047) (-9.101821, -48.04665) (-9.005682, -48.063773) knots 0 0 0 0 1 1 1 1
  spline S217 degree 3 poles (-2.762452, -43.093769) (-2.825615, -43.432923) (-2.920516, -43.762742) (-3.047154, -44.083538) knots 0 0 0 0 1 1 1 1
  spline S218 degree 3 poles (-3.047154, -44.083538) (-3.173481, -44.404334) (-3.329368, -44.710195) (-3.514813, -45.001121) knots 0 0 0 0 1 1 1 1
  spline S219 degree 3 poles (-3.514813, -45.001121) (-3.699948, -45.291735) (-3.911219, -45.562125) (-4.148626, -45.812289) knots 0 0 0 0 1 1 1 1
  spline S220 degree 3 poles (-4.148626, -45.812289) (-4.385723, -46.062454) (-4.6446, -46.287727) (-4.925258, -46.487797) knots 0 0 0 0 1 1 1 1
  spline S221 degree 3 poles (-4.925258, -46.487797) (-5.305483, -46.757564) (-5.714024, -46.97288) (-6.150879, -47.134367) knots 0 0 0 0 1 1 1 1
  spline S222 degree 3 poles (-6.150879, -47.134367) (-6.172659, -47.142457) (-6.193195, -47.152414) (-6.213109, -47.164549) knots 0 0 0 0 1 1 1 1
  spline S223 degree 3 poles (-6.213109, -47.164549) (-6.232712, -47.176683) (-6.251069, -47.190685) (-6.267871, -47.206243) knots 0 0 0 0 1 1 1 1
  spline S224 degree 3 poles (-6.267871, -47.206243) (-6.284985, -47.222111) (-6.300231, -47.239225) (-6.313922, -47.257894) knots 0 0 0 0 1 1 1 1
  spline S225 degree 3 poles (-6.313922, -47.257894) (-6.327301, -47.276563) (-6.338814, -47.296476) (-6.348771, -47.317634) knots 0 0 0 0 1 1 1 1
  spline S226 degree 3 poles (-6.348771, -47.317634) (-6.358416, -47.338482) (-6.365884, -47.360262) (-6.371174, -47.382665) knots 0 0 0 0 1 1 1 1
  spline S227 degree 3 poles (-6.371174, -47.382665) (-6.376463, -47.405068) (-6.379885, -47.428093) (-6.380507, -47.451118) knots 0 0 0 0 1 1 1 1
  spline S228 degree 3 poles (-6.380507, -47.451118) (-6.38144, -47.474143) (-6.380189, -47.497168) (-6.376461, -47.519882) knots 0 0 0 0 1 1 1 1
  spline S229 degree 3 poles (-6.376461, -47.519882) (-6.373036, -47.542907) (-6.367127, -47.564999) (-6.359037, -47.586779) knots 0 0 0 0 1 1 1 1
  spline S230 degree 3 poles (-6.359037, -47.586779) (-6.351254, -47.60856) (-6.341302, -47.629096) (-6.329166, -47.64901) knots 0 0 0 0 1 1 1 1
  spline S231 degree 3 poles (-6.329166, -47.64901) (-6.317032, -47.668612) (-6.30303, -47.68697) (-6.287473, -47.703772) knots 0 0 0 0 1 1 1 1
  spline S232 degree 3 poles (-6.287473, -47.703772) (-6.271915, -47.720885) (-6.25449, -47.736132) (-6.235822, -47.749822) knots 0 0 0 0 1 1 1 1
  spline S233 degree 3 poles (-6.235822, -47.749822) (-6.217152, -47.763202) (-6.19755, -47.775025) (-6.176392, -47.784671) knots 0 0 0 0 1 1 1 1
  spline S234 degree 3 poles (-6.176392, -47.784671) (-6.155545, -47.794317) (-6.133765, -47.801784) (-6.111362, -47.807074) knots 0 0 0 0 1 1 1 1
  spline S235 degree 3 poles (-6.111362, -47.807074) (-6.088959, -47.812675) (-6.066245, -47.815786) (-6.04322, -47.81672) knots 0 0 0 0 1 1 1 1
  spline S236 degree 3 poles (-6.04322, -47.81672) (-6.019884, -47.817651) (-5.997169, -47.816083) (-5.974145, -47.812672) knots 0 0 0 0 1 1 1 1
  spline S237 degree 3 poles (-5.974145, -47.812672) (-5.951431, -47.808936) (-5.929339, -47.803026) (-5.907558, -47.794937) knots 0 0 0 0 1 1 1 1
  spline S238 degree 3 poles (-5.907558, -47.794937) (-5.663617, -47.704703) (-5.42652, -47.598912) (-5.196269, -47.477874) knots 0 0 0 0 1 1 1 1
  spline S239 degree 3 poles (-5.196269, -47.477874) (-4.966018, -47.356526) (-4.74479, -47.221175) (-4.531964, -47.071201) knots 0 0 0 0 1 1 1 1
  spline S240 degree 3 poles (-4.531964, -47.071201) (-4.319137, -46.921538) (-4.1172, -46.758495) (-3.925532, -46.582384) knots 0 0 0 0 1 1 1 1
  spline S241 degree 3 poles (-3.925532, -46.582384) (-3.733863, -46.406584) (-3.554329, -46.218649) (-3.386931, -46.019513) knots 0 0 0 0 1 1 1 1
  spline S242 degree 3 poles (-3.386931, -46.019513) (-3.219532, -45.820066) (-3.065512, -45.610973) (-2.925184, -45.391612) knots 0 0 0 0 1 1 1 1
  spline S243 degree 3 poles (-2.925184, -45.391612) (-2.785166, -45.172251) (-2.659461, -44.9448) (-2.548381, -44.709259) knots 0 0 0 0 1 1 1 1
  spline S244 degree 3 poles (-2.548381, -44.709259) (-2.437611, -44.47403) (-2.342399, -44.232266) (-2.262745, -43.984279) knots 0 0 0 0 1 1 1 1
  spline S245 degree 3 poles (-2.262745, -43.984279) (-2.182779, -43.736292) (-2.119615, -43.484572) (-2.072632, -43.228495) knots 0 0 0 0 1 1 1 1
  spline S246 degree 3 poles (-2.072632, -43.228495) (-2.067965, -43.20547) (-2.065786, -43.182756) (-2.066098, -43.15942) knots 0 0 0 0 1 1 1 1
  spline S247 degree 3 poles (-2.066098, -43.15942) (-2.066098, -43.136394) (-2.068275, -43.113369) (-2.072943, -43.090655) knots 0 0 0 0 1 1 1 1
  spline S248 degree 3 poles (-2.072943, -43.090655) (-2.07761, -43.067941) (-2.084456, -43.04585) (-2.093479, -43.024691) knots 0 0 0 0 1 1 1 1
  spline S249 degree 3 poles (-2.093479, -43.024691) (-2.102502, -43.003222) (-2.113393, -42.982997) (-2.12615, -42.963706) knots 0 0 0 0 1 1 1 1
  spline S250 degree 3 poles (-2.12615, -42.963706) (-2.139218, -42.944415) (-2.153842, -42.926679) (-2.170333, -42.910499) knots 0 0 0 0 1 1 1 1
  spline S251 degree 3 poles (-2.170333, -42.910499) (-2.186824, -42.89432) (-2.204871, -42.879695) (-2.224162, -42.866938) knots 0 0 0 0 1 1 1 1
  spline S252 degree 3 poles (-2.224162, -42.866938) (-2.243454, -42.854181) (-2.263678, -42.843602) (-2.285148, -42.83489) knots 0 0 0 0 1 1 1 1
  spline S253 degree 3 poles (-2.285148, -42.83489) (-2.306617, -42.826178) (-2.328708, -42.819643) (-2.351422, -42.815287) knots 0 0 0 0 1 1 1 1
  line L4 (-2.351422, -42.815287) -> (-2.355778, -42.81465)
  spline S254 degree 3 poles (-2.355778, -42.81465) (-2.378181, -42.810603) (-2.400895, -42.808741) (-2.423609, -42.80905) knots 0 0 0 0 1 1 1 1
  spline S255 degree 3 poles (-2.423609, -42.80905) (-2.446634, -42.809687) (-2.469037, -42.812164) (-2.49144, -42.816824) knots 0 0 0 0 1 1 1 1
  spline S256 degree 3 poles (-2.49144, -42.816824) (-2.513843, -42.821802) (-2.535312, -42.828647) (-2.55647, -42.837671) knots 0 0 0 0 1 1 1 1
  spline S257 degree 3 poles (-2.55647, -42.837671) (-2.577317, -42.846694) (-2.597231, -42.857895) (-2.616211, -42.870653) knots 0 0 0 0 1 1 1 1
  spline S258 degree 3 poles (-2.616211, -42.870653) (-2.635191, -42.883721) (-2.652616, -42.898345) (-2.668485, -42.914525) knots 0 0 0 0 1 1 1 1
  spline S259 degree 3 poles (-2.668485, -42.914525) (-2.684353, -42.931016) (-2.698666, -42.948751) (-2.711423, -42.967732) knots 0 0 0 0 1 1 1 1
  spline S260 degree 3 poles (-2.711423, -42.967732) (-2.723869, -42.987023) (-2.734448, -43.006936) (-2.743161, -43.028406) knots 0 0 0 0 1 1 1 1
  spline S261 degree 3 poles (-2.743161, -43.028406) (-2.751562, -43.049564) (-2.758096, -43.071345) (-2.762452, -43.093769) knots 0 0 0 0 1 1 1 1
  spline S262 degree 3 poles (-4.132447, -42.767061) (-4.175074, -43.02376) (-4.242283, -43.273614) (-4.334072, -43.517245) knots 0 0 0 0 1 1 1 1
  spline S263 degree 3 poles (-4.334072, -43.517245) (-4.425861, -43.760564) (-4.540676, -43.992682) (-4.677893, -44.213599) knots 0 0 0 0 1 1 1 1
  spline S264 degree 3 poles (-4.677893, -44.213599) (-4.815422, -44.434516) (-4.973175, -44.639875) (-5.150842, -44.829677) knots 0 0 0 0 1 1 1 1
  spline S265 degree 3 poles (-5.150842, -44.829677) (-5.328819, -45.019478) (-5.523289, -45.189989) (-5.734559, -45.341519) knots 0 0 0 0 1 1 1 1
  spline S266 degree 3 poles (-5.734559, -45.341519) (-5.942719, -45.489315) (-6.163325, -45.61502) (-6.396376, -45.718633) knots 0 0 0 0 1 1 1 1
  spline S267 degree 3 poles (-6.396376, -45.718633) (-6.629739, -45.822246) (-6.87057, -45.901589) (-7.119801, -45.956663) knots 0 0 0 0 1 1 1 1
  spline S268 degree 3 poles (-7.119801, -45.956663) (-7.368721, -46.012048) (-7.620753, -46.041918) (-7.875585, -46.046586) knots 0 0 0 0 1 1 1 1
  spline S269 degree 3 poles (-7.875585, -46.046586) (-8.130728, -46.051253) (-8.383693, -46.030717) (-8.63448, -45.984667) knots 0 0 0 0 1 1 1 1
  spline S270 degree 3 poles (-8.63448, -45.984667) (-8.906426, -45.936127) (-9.16997, -45.858962) (-9.425424, -45.753482) knots 0 0 0 0 1 1 1 1
  spline S271 degree 3 poles (-9.425424, -45.753482) (-9.680879, -45.648313) (-9.922331, -45.517008) (-10.149782, -45.359877) knots 0 0 0 0 1 1 1 1
  spline S272 degree 3 poles (-10.149782, -45.359877) (-10.376922, -45.202746) (-10.585081, -45.023212) (-10.77395, -44.821587) knots 0 0 0 0 1 1 1 1
  spline S273 degree 3 poles (-10.77395, -44.821587) (-10.962818, -44.61965) (-11.128039, -44.399978) (-11.269923, -44.162571) knots 0 0 0 0 1 1 1 1
  spline S274 degree 3 poles (-11.269923, -44.162571) (-11.281436, -44.142035) (-11.294815, -44.122743) (-11.310061, -44.104697) knots 0 0 0 0 1 1 1 1
  spline S275 degree 3 poles (-11.310061, -44.104697) (-11.325308, -44.086961) (-11.342421, -44.07047) (-11.360779, -44.056157) knots 0 0 0 0 1 1 1 1
  spline S276 degree 3 poles (-11.360779, -44.056157) (-11.379448, -44.041533) (-11.399362, -44.028776) (-11.42052, -44.018508) knots 0 0 0 0 1 1 1 1
  spline S277 degree 3 poles (-11.42052, -44.018508) (-11.441367, -44.007929) (-11.463459, -43.999528) (-11.486173, -43.993305) knots 0 0 0 0 1 1 1 1
  spline S278 degree 3 poles (-11.486173, -43.993305) (-11.508887, -43.987084) (-11.532223, -43.983348) (-11.555559, -43.981792) knots 0 0 0 0 1 1 1 1
  spline S279 degree 3 poles (-11.555559, -43.981792) (-11.579206, -43.98055) (-11.602543, -43.981474) (-11.625879, -43.984595) knots 0 0 0 0 1 1 1 1
  spline S280 degree 3 poles (-11.625879, -43.984595) (-11.649214, -43.98802) (-11.67224, -43.993307) (-11.694332, -44.001397) knots 0 0 0 0 1 1 1 1
  spline S281 degree 3 poles (-11.694332, -44.001397) (-11.716735, -44.009171) (-11.737893, -44.019133) (-11.758118, -44.031268) knots 0 0 0 0 1 1 1 1
  spline S282 degree 3 poles (-11.758118, -44.031268) (-11.778343, -44.043402) (-11.797323, -44.057404) (-11.814436, -44.073273) knots 0 0 0 0 1 1 1 1
  spline S283 degree 3 poles (-11.814436, -44.073273) (-11.831861, -44.089141) (-11.847729, -44.106877) (-11.86142, -44.125857) knots 0 0 0 0 1 1 1 1
  spline S284 degree 3 poles (-11.86142, -44.125857) (-11.875422, -44.144837) (-11.887245, -44.165373) (-11.897202, -44.186843) knots 0 0 0 0 1 1 1 1
  spline S285 degree 3 poles (-11.897202, -44.186843) (-11.906848, -44.208312) (-11.914626, -44.230404) (-11.919916, -44.253429) knots 0 0 0 0 1 1 1 1
  spline S286 degree 3 poles (-11.919916, -44.253429) (-11.925206, -44.276454) (-11.928317, -44.29979) (-11.928939, -44.323438) knots 0 0 0 0 1 1 1 1
  spline S287 degree 3 poles (-11.928939, -44.323438) (-11.929576, -44.346774) (-11.928007, -44.370421) (-11.923961, -44.393758) knots 0 0 0 0 1 1 1 1
  spline S288 degree 3 poles (-11.923961, -44.393758) (-11.919915, -44.416783) (-11.913693, -44.439497) (-11.904981, -44.461588) knots 0 0 0 0 1 1 1 1
  spline S289 degree 3 poles (-11.904981, -44.461588) (-11.89658, -44.483369) (-11.88569, -44.504527) (-11.872932, -44.52413) knots 0 0 0 0 1 1 1 1
  spline S290 degree 3 poles (-11.872932, -44.52413) (-11.789544, -44.664147) (-11.698688, -44.799186) (-11.600676, -44.929247) knots 0 0 0 0 1 1 1 1
  spline S291 degree 3 poles (-11.600676, -44.929247) (-11.502664, -45.059308) (-11.398117, -45.183768) (-11.286725, -45.302939) knots 0 0 0 0 1 1 1 1
  spline S292 degree 3 poles (-11.286725, -45.302939) (-11.175333, -45.421798) (-11.05803, -45.534435) (-10.934814, -45.640848) knots 0 0 0 0 1 1 1 1
  spline S293 degree 3 poles (-10.934814, -45.640848) (-10.811599, -45.747261) (-10.682782, -45.846829) (-10.548988, -45.939241) knots 0 0 0 0 1 1 1 1
  spline S294 degree 3 poles (-10.548988, -45.939241) (-10.414882, -46.031964) (-10.27642, -46.117219) (-10.133602, -46.195007) knots 0 0 0 0 1 1 1 1
  spline S295 degree 3 poles (-10.133602, -46.195007) (-9.990473, -46.272794) (-9.84361, -46.342492) (-9.693013, -46.404722) knots 0 0 0 0 1 1 1 1
  spline S296 degree 3 poles (-9.693013, -46.404722) (-9.542728, -46.466641) (-9.389331, -46.52047) (-9.232822, -46.566209) knots 0 0 0 0 1 1 1 1
  spline S297 degree 3 poles (-9.232822, -46.566209) (-9.076625, -46.611948) (-8.918249, -46.648975) (-8.758007, -46.677601) knots 0 0 0 0 1 1 1 1
  spline S298 degree 3 poles (-8.758007, -46.677601) (-8.461481, -46.731741) (-8.162465, -46.755388) (-7.861272, -46.749476) knots 0 0 0 0 1 1 1 1
  spline S299 degree 3 poles (-7.861272, -46.749476) (-7.559767, -46.743567) (-7.261996, -46.707471) (-6.967959, -46.641818) knots 0 0 0 0 1 1 1 1
  spline S300 degree 3 poles (-6.967959, -46.641818) (-6.67361, -46.576166) (-6.388908, -46.481887) (-6.113229, -46.359294) knots 0 0 0 0 1 1 1 1
  spline S301 degree 3 poles (-6.113229, -46.359294) (-5.837861, -46.23639) (-5.577428, -46.08766) (-5.33162, -45.912793) knots 0 0 0 0 1 1 1 1
  spline S302 degree 3 poles (-5.33162, -45.912793) (-5.081766, -45.733882) (-4.851514, -45.532568) (-4.641177, -45.308539) knots 0 0 0 0 1 1 1 1